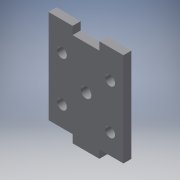
# Autodesk Inventor part: Camera mount side bars
Saved by Autodesk Inventor 2018 (Build 220112000, 112)
## iProperties
Created: 2018-06-25
Part Number: Camera mount side bars
Material: Generic
Document SubType Name: Modeling
Designer: Ajith Thomas
Density: 1 g/cm^3
Appearance: Default
Author: Ajith Thomas
Autodesk Inventor part; units mm, degrees
ref_plane "YZ Plane" through (0, 0, 0) normal (1, 0, 0) x (0, 1, 0)
ref_plane "XZ Plane" through (0, 0, 0) normal (0, 1, 0) x (-1, 0, 0)
ref_plane "XY Plane" through (0, 0, 0) normal (0, 0, 1) x (1, 0, 0)
sketch "Sketch1" plane through (0, 0, 0) normal (0, 0, 1) x (1, 0, 0)
  line L0 (-9, 0) -> (0, 0) construction
  line L1 (-19, 0) -> (-9, 0) construction
  line L2 (-28, 0) -> (-19, 0) construction
  line L3 (0, 0) -> (-28, 0)
  line L4 (-28, 0) -> (-28, -35)
  line L5 (-28, -35) -> (0, -35)
  line L6 (0, -35) -> (0, 0)
  line L7 (-19, 0) -> (-9, 0) projected
  line L8 (-19, 0) -> (-19, -3) projected
  line L9 (-9, -3) -> (-19, -3) projected
  line L10 (-9, 0) -> (-9, -3) projected
  dimension "d0" = 35
  constraints: 8 end point, 2 parallel, 1 horizontal, 1 perpendicular
  measures "d0" distance of L4.end L3.end
extrude "Extrusion1" add sketch "Sketch1" along normal blind 3 contours L6 L5 L4 L3 L8 L9 L10
sketch "Sketch2" plane through (0, 0, 0) normal (0, 0, -1) x (-1, 0, 0)
  arc A0 (6.85, -9.25) -> (3.15, -9.25) centre (5, -9.25) ccw construction
  line L0 (6.85, -9.25) -> (6.85, -12.05) construction
  arc A1 (3.15, -12.05) -> (6.85, -12.05) centre (5, -12.05) ccw construction
  line L1 (3.15, -12.05) -> (3.15, -9.25) construction
  line L2 (21.15, -12.05) -> (21.15, -9.25) construction
  arc A2 (21.15, -12.05) -> (24.85, -12.05) centre (23, -12.05) ccw construction
  line L3 (24.85, -9.25) -> (24.85, -12.05) construction
  arc A3 (24.85, -9.25) -> (21.15, -9.25) centre (23, -9.25) ccw construction
  line L4 (5, -12.05) -> (5, -9.25) construction
  line L5 (5, -10.65) -> (3.15, -10.65) construction
  line L6 (23, -12.05) -> (23, -9.25) construction
  line L7 (23, -10.65) -> (21.15, -10.65) construction
  circle A4 centre (5, -10.65) radius 1.85
  circle A5 centre (23, -10.65) radius 1.85
  point P0 (0, 0)
  constraints: 8 end point, 4 midpoint, 2 coincident, 2 horizontal alignment, 2 vertical, 4 other
extrude "Extrusion2" cut sketch "Sketch2" against normal blind 6.175
sketch "Sketch3" plane through (0, 0, 3) normal (0, 0, 1) x (1, 0, 0)
  line L0 (-9, -3) -> (-19, -3) projected
  line L1 (-28, -35) -> (0, -35) projected
  line L2 (-14, -3) -> (-14, -35) construction
  line L3 (-28, -35) -> (0, -35) construction
  line L4 (-14, -19) -> (0, -19) construction
  line L5 (0, -35) -> (0, 0) construction
  circle A0 centre (-14, -19) radius 2
  dimension "d5" = 4
  constraints: 4 end point, 3 midpoint, 1 centre point, 1 coincident, 1 perpendicular, 1 point on line
  measures "d5" diameter of A0
extrude "Extrusion3" cut sketch "Sketch3" against normal blind 6.175
sketch "Sketch4" plane through (-28, -35, 0) normal (0, -1, 0) x (1, 0, 0)
  line L0 (9, 3) -> (19, 3) projected
  line L1 (19, 3) -> (19, 0) projected
  line L2 (9, 0) -> (19, 0) projected
  line L3 (9, 0) -> (9, 3) projected
  point P0 (28, 0)
extrude "Extrusion4" add sketch "Sketch4" along normal blind 3
sketch "Sketch5" plane through (0, 0, 0) normal (0, 0, -1) x (-1, 0, 0)
  arc A0 (6.85, -25.95) -> (3.15, -25.95) centre (5, -25.95) ccw construction
  line L0 (6.85, -25.95) -> (6.85, -28.75) construction
  arc A1 (3.15, -28.75) -> (6.85, -28.75) centre (5, -28.75) ccw construction
  line L1 (3.15, -28.75) -> (3.15, -25.95) construction
  arc A2 (1, -20.4) -> (0, -21.4) centre (1, -21.4) ccw construction
  line L2 (0, -21.4) -> (0, -34) construction
  line L3 (0, -34) -> (10, -34) construction
  line L4 (10, -34) -> (10, -21.4) construction
  arc A3 (10, -21.4) -> (9, -20.4) centre (9, -21.4) ccw construction
  line L5 (9, -20.4) -> (1, -20.4) construction
  arc A4 (24.85, -25.95) -> (21.15, -25.95) centre (23, -25.95) ccw construction
  line L6 (24.85, -25.95) -> (24.85, -28.75) construction
  arc A5 (21.15, -28.75) -> (24.85, -28.75) centre (23, -28.75) ccw construction
  line L7 (21.15, -28.75) -> (21.15, -25.95) construction
  arc A6 (19, -20.4) -> (18, -21.4) centre (19, -21.4) ccw construction
  line L8 (18, -21.4) -> (18, -34) construction
  line L9 (18, -34) -> (28, -34) construction
  line L10 (28, -34) -> (28, -21.4) construction
  arc A7 (28, -21.4) -> (27, -20.4) centre (27, -21.4) ccw construction
  line L11 (27, -20.4) -> (19, -20.4) construction
  line L12 (5, -28.75) -> (5, -25.95) construction
  line L13 (23, -28.75) -> (23, -25.95) construction
  circle A8 centre (5, -27.35) radius 1.85
  circle A9 centre (23, -27.35) radius 1.85
  point P0 (0, 0)
  constraints: 4 end point, 2 centre point, 2 midpoint, 2 vertical, 1 tangent
extrude "Extrusion5" cut sketch "Sketch5" against normal blind 3
body "Solid1"
